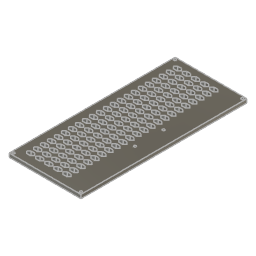
Couvercle Boite (Autodesk Fusion 360 design; units mm, degrees)
Autodesk Fusion 360 part; units mm, degrees
note: some values were not read from the file. Set by a fixed rule: which sketch regions a step uses.
sketch "Esquisse1" plane through (0, 0, 0) normal (0, 0, 1) x (1, 0, 0)
  line L0 (0, 0) -> (79, 0)
  line L1 (79, 0) -> (79, 201)
  line L2 (79, 201) -> (0, 201)
  line L3 (0, 201) -> (0, 0)
  line L4 (-7, 208) -> (86, 208)
  line L5 (86, 208) -> (86, -7)
  line L6 (86, -7) -> (-7, -7)
  line L7 (-7, -7) -> (-7, 208)
  dimension "d1" = 201
  dimension "d2" = 79
  dimension "d3" = 7
  dimension "d4" = 7
  dimension "d5" = 7
  dimension "d6" = 7
  constraint horizontal L0
  constraint vertical L1
  constraint horizontal L2
  constraint vertical L3
  constraint coincident L0.start L3.end
  constraint horizontal L4
  constraint vertical L5
  constraint horizontal L6
  constraint vertical L7
  measures "d1" distance of L0.start L2.end
  measures "d2" distance of L1.end L2.end
  measures "d3" distance of L3 L7
  measures "d4" distance of L2 L4
  measures "d5" distance of L1 L5
  measures "d6" distance of L0 L6
extrude "Extrusion1" add sketch "Esquisse1" along normal blind 5 from surface at 5
extrude "Extrusion2" add sketch "Esquisse1" along normal blind 5 from surface at 5 contours L0 L1 L2 L3
sketch "Esquisse2" plane through (0, 0, 10) normal (0, 0, 1) x (-1, 0, 0)
  circle A0 centre (4, 4) radius 1.55
  line L0 (7, -208) -> (7, 7)
  line L1 (7, 7) -> (-86, 7)
  circle A1 centre (4, -205) radius 1.55
  line L2 (-86, -208) -> (7, -208)
  circle A2 centre (-83, -205) radius 1.55
  line L3 (-86, 7) -> (-86, -208)
  circle A3 centre (-83, 4) radius 1.55
  dimension "d99" = 3.1
  dimension "d100" = 3
  dimension "d101" = 3
  dimension "d102" = 3.1
  dimension "d103" = 3
  dimension "d104" = 3
  dimension "d105" = 3.1
  dimension "d106" = 3
  dimension "d107" = 3
  dimension "d108" = 3.1
  dimension "d109" = 3
  dimension "d110" = 3
  measures "d99" diameter of A0
  measures "d100" distance of A0.centre L0
  measures "d101" distance of A0.centre L1
  measures "d102" diameter of A1
  measures "d103" distance of A1.centre L2
  measures "d104" distance of L0 A1.centre
  measures "d105" diameter of A2
  measures "d106" distance of L2 A2.centre
  measures "d107" distance of A2.centre L3
  measures "d108" diameter of A3
  measures "d109" distance of L3 A3.centre
  measures "d110" distance of L1 A3.centre
extrude "Extrusion3" cut sketch "Esquisse2" against normal blind 18 contours A0 | A1 | A2 | A3
sketch "Esquisse5" plane through (0, 0, 10) normal (0, 0, 1) x (-1, 0, 0)
  line L0 (7, 7) -> (-86, 7)
  line L1 (-86, 7) -> (-86, -208)
  line L2 (-86, -208) -> (7, -208)
  line L3 (7, -208) -> (7, 7)
  circle A0 centre (-83, -205) radius 1.55
  circle A1 centre (4, 4) radius 1.55
  circle A2 centre (4, -205) radius 1.55
  circle A3 centre (-83, 4) radius 1.55
  line L4 (-55.5, -178.3787) -> (-55.5, -208)
  line L5 (-55.5, -178.3787) -> (-55.5, 7)
  line L6 (-63.7426, -21.3787) -> (-63.7426, 7)
  line L7 (-63.7426, -21.3787) -> (-63.7426, -208)
  line L8 (-5.5, -21.3787) -> (-5.5, 7)
  line L9 (-5.5, -21.3787) -> (-5.5, -208)
  line L10 (-13.7426, -21.3787) -> (-13.7426, 7)
  line L11 (-13.7426, -21.3787) -> (-13.7426, -208)
  line L12 (-65.5, -21.3787) -> (-65.5, 7)
  line L13 (-65.5, -21.3787) -> (-65.5, -208)
  line L14 (-73.7426, -21.3787) -> (-73.7426, 7)
  line L15 (-73.7426, -21.3787) -> (-73.7426, -208)
  constraint coincident L2 L4.end
  constraint perpendicular L2 L4
  constraint coincident L0 L5.end
  constraint perpendicular L0 L5
  constraint coincident L0 L6.end
  constraint perpendicular L0 L6
  constraint coincident L2 L7.end
  constraint perpendicular L2 L7
  constraint coincident L0 L8.end
  constraint perpendicular L0 L8
  constraint coincident L2 L9.end
  constraint perpendicular L2 L9
  constraint coincident L0 L10.end
  constraint perpendicular L0 L10
  constraint coincident L2 L11.end
  constraint perpendicular L2 L11
  constraint coincident L0 L12.end
  constraint perpendicular L0 L12
  constraint coincident L2 L13.end
  constraint perpendicular L2 L13
  constraint coincident L0 L14.end
  constraint perpendicular L0 L14
  constraint coincident L2 L15.end
  constraint perpendicular L2 L15
sketch "Esquisse4" plane through (0, 0, 10) normal (0, 0, 1) x (-1, 0, 0)
  circle A0 centre (-67, -82) radius 1.55
  circle A1 centre (-67, -119) radius 1.55
  line L0 (7, 7) -> (-86, 7)
  line L1 (-86, 7) -> (-86, -208)
  line L2 (-86, -208) -> (7, -208)
  line L3 (7, -208) -> (7, 7)
  circle A2 centre (-83, -205) radius 1.55
  circle A3 centre (4, 4) radius 1.55
  circle A4 centre (4, -205) radius 1.55
  circle A5 centre (-83, 4) radius 1.55
  dimension "d60" = 3.1
  dimension "d61" = 3.1
  dimension "d115" = 19
  dimension "d116" = 19
  dimension "d117" = 89
  dimension "d119" = 37
  measures "d60" diameter of A0
  measures "d61" diameter of A1
  measures "d115" distance of A0.centre L1
  measures "d116" distance of A1.centre L1
  measures "d117" distance of A0.centre L0
  measures "d119" distance of A0.centre A1.centre
extrude "Extrusion10" add sketch "Esquisse5" against normal blind 5 contours L0 L2 L4 L5 L10 L11 | L0 L2 L4 L5 L6 L7 | L0 L2 L6 L7 L12 L13 | L0 L2 L12 L13 L14 L15
extrude "Extrusion5" cut sketch "Esquisse4" against normal blind 5 contours A0 | A1
sketch "Esquisse6" plane through (0, 0, 10) normal (0, 0, 1) x (-1, 0, 0)
  circle A0 centre (-67, -82) radius 1.55
  circle A1 centre (-67, -119) radius 1.55
  circle A2 centre (4, 4) radius 1.55
  circle A3 centre (4, -205) radius 1.55
  line L0 (7, 7) -> (-86, 7)
  line L1 (-86, 7) -> (-86, -208)
  line L2 (-86, -208) -> (7, -208)
  line L3 (7, -208) -> (7, 7)
  circle A4 centre (-83, -205) radius 1.55
  circle A5 centre (-83, 4) radius 1.55
  line L4 (-86, -208) -> (7, -208)
  line L5 (7, -208) -> (7, 7)
  line L6 (-86, 7) -> (-86, -208)
  line L7 (7, 7) -> (-86, 7)
  line L8 (7, 7) -> (-0.0711, -0.0711)
  line L9 (-86, -208) -> (-78.9289, -200.9289)
  line L10 (-78.9289, -200.9289) -> (-0.0711, -200.9289)
  line L11 (-0.0711, -200.9289) -> (-0.0711, -0.0711)
  line L12 (-0.0711, -0.0711) -> (-78.9289, -0.0711)
  line L13 (-78.9289, -0.0711) -> (-78.9289, -200.9289)
  line L14 (-4.3137, -200.9289) -> (-0.0711, -196.6863)
  line L15 (-0.0711, -196.6863) -> (-4.3137, -192.4437)
  line L16 (-10.3137, -200.9289) -> (-14.5563, -196.6863)
  line L17 (-14.5563, -196.6863) -> (-10.3137, -192.4437)
  line L18 (-4.3137, -192.4437) -> (-10.3137, -192.4437)
  line L19 (-0.0711, -196.6863) -> (-2.0711, -196.6863)
  line L20 (-14.5563, -196.6863) -> (-12.5563, -196.6863)
  line L21 (-2.0711, -196.6863) -> (-4.8995, -199.5147)
  line L22 (-2.0711, -196.6863) -> (-4.8995, -193.8579)
  line L23 (-12.5563, -196.6863) -> (-9.7279, -193.8579)
  line L24 (-12.5563, -196.6863) -> (-9.7279, -199.5147)
  line L25 (-4.8995, -199.5147) -> (-9.7279, -199.5147)
  line L26 (-4.8995, -193.8579) -> (-9.7279, -193.8579)
  point P0 (-10.3137, -200.9289)
  dimension "d122" = 45
  dimension "d123" = 10
  dimension "d124" = 45
  dimension "d126" = 10
  dimension "d127" = 45
  dimension "d130" = 6
  dimension "d131" = 6
  dimension "d132" = 6
  dimension "d133" = 45
  dimension "d134" = 6
  dimension "d135" = 6
  dimension "d136" = 2
  dimension "d137" = 2
  dimension "d138" = 135
  dimension "d139" = 4
  dimension "d140" = 4
  dimension "d141" = 4
  dimension "d142" = 4
  constraint coincident L0.start L3.end
  constraint coincident L1.end L2.start
  constraint horizontal L10
  constraint vertical L11
  constraint horizontal L12
  constraint vertical L13
  constraint coincident L10 L14.start
  constraint coincident L11 L14.end
  constraint perpendicular L14 L15
  constraint coincident L10 P0
  constraint coincident P0 L16.start
  constraint perpendicular L16 L17
  constraint perpendicular L11 L19
  constraint horizontal L20
  constraint perpendicular L21 L22
  constraint parallel L17 L23
  constraint perpendicular L23 L24
  measures "d122" angle of L7 L8
  measures "d123" distance of L0.start L8.end
  measures "d124" angle of L4 L9
  measures "d126" distance of L1.end L9.end
  measures "d127" angle of L10 L14
  measures "d130" distance of L14.start L14.end
  measures "d131" distance of L14.end L15.end
  measures "d132" distance of L14.start P0
  measures "d133" angle of L10 L16
  measures "d134" distance of P0 L16.end
  measures "d135" distance of L16.end L17.end
  measures "d136" distance of L14.end L19.end
  measures "d137" distance of L16.end L20.end
  measures "d138" angle of L19 L21
  measures "d139" distance of L19.end L21.end
  measures "d140" distance of L19.end L22.end
  measures "d141" distance of L20.end L23.end
  measures "d142" distance of L20.end L24.end
extrude "Extrusion11" cut sketch "Esquisse6" against normal blind 10 contours L21 L22 L23 L24 L25 L26
pattern_linear "Réseau R4" count 5 spacing 11.75 along (1, 0, 0) of "Extrusion11"
pattern_linear "Réseau R5" count 22 spacing 9.0476 along (0, -1, 0) of "Extrusion11", "Réseau R4"
component "Couvercle Boite v35" placed x (1, 0, 0) y (0, 1, 0) z (0, 0, 1) at (0, 0, 0)
